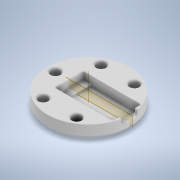
# Autodesk Inventor part: hmmb
Saved by Autodesk Inventor 2021 (Build 250183000, 183)
## iProperties
Created: 2020-07-09
Part Number: hmmb
Material: Generic
Document SubType Name: Modeling
Designer: andre
Density: 1 g/cm^3
Appearance: Default
Author: andre
## iProperties of the stored document _3DPrint.ipt
Created: 2020-07-09
Part Number: _3DPrint
Material: Generic
Document SubType Name: Modeling
Designer: andre
Density: 1 g/cm^3
Appearance: Default
Author: andre
Autodesk Inventor part; units mm, degrees
ref_plane "YZ Plane" through (0, 0, 0) normal (1, 0, 0) x (0, 1, 0)
ref_plane "XZ Plane" through (0, 0, 0) normal (0, 1, 0) x (-1, 0, 0)
ref_plane "XY Plane" through (0, 0, 0) normal (0, 0, 1) x (1, 0, 0)
sketch "Sketch1" plane through (0, 0, 0) normal (0, 1, 0) x (-1, 0, 0)
  circle A0 centre (0, 0) radius 26
  dimension "d0" = 52
  constraints: 1 centre point
  measures "d0" diameter of A0
extrude "Extrusion1" add sketch "Sketch1" along normal blind 8
chamfer "Chamfer2" distance 1.6 angle 45 1 edges at (26, 0, 0)
sketch "Sketch2" plane through (0, 8, 0) normal (0, 1, 0) x (1, 0, 0)
  line L0 (-12.4, -8.99) -> (23.96, -8.99)
  line L1 (23.96, -8.99) -> (23.96, 8.99)
  line L2 (23.96, 8.99) -> (-12.4, 8.99)
  line L3 (-12.4, 8.99) -> (-12.4, -8.99)
  point P0 (0, 0)
  dimension "d5" = 36.36
  dimension "d6" = 17.98
  dimension "d7" = 8.99
  dimension "d8" = 12.4
  constraints: 8 end point, 2 parallel, 1 horizontal, 1 perpendicular
  measures "d5" distance of L2.end L1.end
  measures "d6" distance of L1.end L0.end
  measures "d7" distance from line of point (0, 0) L2
  measures "d8" distance from line of point (0, 0) L3
extrude "Extrusion2" cut sketch "Sketch2" against normal blind 4.8
sketch "Sketch3" plane through (23.96, 8, -8.99) normal (-1, 0, 0) x (0, 0, 1)
  line L0 (4, 0) -> (13.98, 0)
  line L1 (13.98, 0) -> (13.98, -3.8)
  line L2 (13.98, -3.8) -> (4, -3.8)
  line L3 (4, -3.8) -> (4, 0)
  line L4 (0, 0) -> (17.98, 0) projected
  line L5 (0, -4.8) -> (17.98, -4.8) projected
  line L6 (0, 0) -> (0, -4.8) projected
  line L7 (17.98, 0) -> (17.98, -4.8) projected
  point P0 (8.99, -8)
  dimension "d11" = 0
  dimension "d14" = 4
  dimension "d44" = 4
  dimension "d47" = 1
  constraints: 8 end point, 2 parallel, 1 horizontal, 1 perpendicular
  measures "d11" distance between parallel lines of L4 L0
  measures "d14" distance between parallel lines of L7 L1
  measures "d44" distance between parallel lines of L6 L3
  measures "d47" distance between parallel lines of L5 L2
extrude "Extrusion3" cut sketch "Sketch3" against normal through all contours L0 L1 L2 L3
ref_plane "Work Plane1" through (-12.4, 8, 0) normal (0, 0, 1) x (1, 0, 0)
sketch "Sketch7" plane through (0, 3.2, 0) normal (0, 1, 0) x (1, 0, 0)
  line L0 (-7.4, 8.99) -> (21.36, 8.99)
  line L1 (21.36, 8.99) -> (21.36, -8.99)
  line L2 (21.36, -8.99) -> (-7.4, -8.99)
  line L3 (-7.4, -8.99) -> (-7.4, 8.99)
  line L4 (36.4, 0) -> (-36.4, 0) projected
  line L5 (-12.4, -8.99) -> (-12.4, 8.99) projected
  line L6 (23.96, -8.99) -> (-12.4, -8.99) projected
  line L7 (23.96, -4.99) -> (23.96, -8.99) projected
  line L8 (-12.4, 8.99) -> (23.96, 8.99) projected
  point P0 (0, 0)
  dimension "d31" = 5
  dimension "d98" = 2.6
  dimension "d99" = 0
  dimension "d100" = 0
  constraints: 8 end point, 2 parallel, 1 horizontal, 1 perpendicular
  measures "d31" distance between parallel lines of L5 L3
  measures "d98" distance between parallel lines of L7 L1
  measures "d99" distance between parallel lines of L6 L2
  measures "d100" distance between parallel lines of L8 L0
extrude "Extrusion5" cut sketch "Sketch7" against normal blind 1.6 contours L0 L1 L4 L3 | L4 L1 L2 L3
sketch "Sketch4" plane through (0, 8, 0) normal (0, 1, 0) x (1, 0, 0)
  circle A0 centre (-21, 0) radius 2.8
  arc A1 (25.5167, 4.99) -> (25.5167, -4.99) centre (0, 0) ccw projected
  point P0 (24.6995, 8.12)
  point P1 (24.6995, -8.12)
  dimension "d17" = 5.6
  dimension "d23" = 21
  constraints: 1 centre point
  measures "d17" diameter of A0
  measures "d23" distance of A0.centre A1.centre
extrude "Extrusion4" cut sketch "Sketch4" against normal blind 5.2
fillet "Fillet4" radius 1 1 edges at (-23.8, 8, 0)
pattern_circular "Circular Pattern2" count 5 over 240 about axis through (0, 8, 0) along (0, 1, 0) of "Extrusion4", "Fillet4" both ways yes
fillet "Fillet7" radius 0.8 4 edges at (23.96, 5.6, -8.99) (23.96, 5.6, 8.99) (-12.4, 5.6, 8.99) (-12.4, 5.6, -8.99) curvature continuous yes
sketch "Sketch12" plane through (0, 0, 0) normal (0, -1, 0) x (1, 0, 0)
  line L0 (12.3547, 15) -> (12.3547, -15) construction
  line L1 (12.3547, -15) -> (-12.3547, -15) construction
  line L2 (-12.3547, -15) -> (-12.3547, 15) construction
  line L3 (-12.3547, 15) -> (12.3547, 15) construction
  spline S0 degree 2 poles (-6.9887, 11.414) (-7, 11.0864) (-6.7175, 10.6231) (-6.3785, 10.3858) knots 0 0 0 1 2 2 2
  line L4 (-6.3785, 10.3858) -> (-1.8136, 7.1542)
  line L5 (-1.8136, 7.1542) -> (-1.8136, 7.0864)
  line L6 (-1.8136, 7.0864) -> (-6.3898, 3.8321)
  spline S1 degree 2 poles (-6.3898, 3.8321) (-6.7062, 3.6061) (-7, 3.109) (-6.9887, 2.77) knots 0 0 0 1 2 2 2
  spline S2 degree 2 poles (-6.9887, 2.77) (-6.9774, 2.2615) (-6.3672, 1.5948) (-5.8814, 1.5835) knots 0 0 0 1 2 2 2
  spline S3 degree 2 poles (-5.8814, 1.5835) (-5.6554, 1.5835) (-5.2373, 1.7304) (-5.0339, 1.8886) knots 0 0 0 1 2 2 2
  line L7 (-5.0339, 1.8886) -> (-0.0395, 5.527)
  line L8 (-0.0395, 5.527) -> (0.0282, 5.527)
  line L9 (0.0282, 5.527) -> (5.113, 1.7756)
  spline S4 degree 2 poles (5.113, 1.7756) (5.3277, 1.6174) (5.7345, 1.4705) (5.9492, 1.4818) knots 0 0 0 1 2 2 2
  spline S5 degree 2 poles (5.9492, 1.4818) (6.4011, 1.4931) (6.9887, 2.1598) (6.9887, 2.657) knots 0 0 0 1 2 2 2
  spline S6 degree 2 poles (6.9887, 2.657) (7, 2.996) (6.7062, 3.4479) (6.3898, 3.6626) knots 0 0 0 1 2 2 2
  line L10 (6.3898, 3.6626) -> (1.7006, 6.9169)
  line L11 (1.7006, 6.9169) -> (1.7006, 6.9847)
  line L12 (1.7006, 6.9847) -> (6.3107, 10.1485)
  spline S7 degree 2 poles (6.3107, 10.1485) (6.6723, 10.3971) (7, 10.9056) (6.9887, 11.2446) knots 0 0 0 1 2 2 2
  spline S8 degree 2 poles (6.9887, 11.2446) (6.9887, 11.7982) (6.3559, 12.4762) (5.8588, 12.4875) knots 0 0 0 1 2 2 2
  spline S9 degree 2 poles (5.8588, 12.4875) (5.6328, 12.4875) (5.2034, 12.3519) (4.9548, 12.1598) knots 0 0 0 1 2 2 2
  line L13 (4.9548, 12.1598) -> (0.0847, 8.6231)
  line L14 (0.0847, 8.6231) -> (0.0169, 8.6231)
  line L15 (0.0169, 8.6231) -> (-5.0791, 12.2728)
  spline S10 degree 2 poles (-5.0791, 12.2728) (-5.3051, 12.431) (-5.7232, 12.5892) (-5.9266, 12.5892) knots 0 0 0 1 2 2 2
  spline S11 degree 2 poles (-5.9266, 12.5892) (-6.3898, 12.5779) (-6.9774, 11.9225) (-6.9887, 11.414) knots 0 0 0 1 2 2 2
  spline S12 degree 2 poles (-6.9887, -2.6344) (-7, -2.9621) (-6.7175, -3.4253) (-6.3785, -3.6626) knots 0 0 0 1 2 2 2
  line L16 (-6.3785, -3.6626) -> (-1.8136, -6.8943)
  line L17 (-1.8136, -6.8943) -> (-1.8136, -6.9621)
  line L18 (-1.8136, -6.9621) -> (-6.3898, -10.2163)
  spline S13 degree 2 poles (-6.3898, -10.2163) (-6.7062, -10.4423) (-7, -10.9395) (-6.9887, -11.2785) knots 0 0 0 1 2 2 2
  spline S14 degree 2 poles (-6.9887, -11.2785) (-6.9774, -11.7869) (-6.3672, -12.4536) (-5.8814, -12.4649) knots 0 0 0 1 2 2 2
  spline S15 degree 2 poles (-5.8814, -12.4649) (-5.6554, -12.4649) (-5.2373, -12.318) (-5.0339, -12.1598) knots 0 0 0 1 2 2 2
  line L19 (-5.0339, -12.1598) -> (-0.0395, -8.5214)
  line L20 (-0.0395, -8.5214) -> (0.0282, -8.5214)
  line L21 (0.0282, -8.5214) -> (5.113, -12.2728)
  spline S16 degree 2 poles (5.113, -12.2728) (5.3277, -12.431) (5.7345, -12.5779) (5.9492, -12.5666) knots 0 0 0 1 2 2 2
  spline S17 degree 2 poles (5.9492, -12.5666) (6.4011, -12.5553) (6.9887, -11.8886) (6.9887, -11.3914) knots 0 0 0 1 2 2 2
  spline S18 degree 2 poles (6.9887, -11.3914) (7, -11.0525) (6.7062, -10.6005) (6.3898, -10.3858) knots 0 0 0 1 2 2 2
  line L22 (6.3898, -10.3858) -> (1.7006, -7.1316)
  line L23 (1.7006, -7.1316) -> (1.7006, -7.0638)
  line L24 (1.7006, -7.0638) -> (6.3107, -3.8999)
  spline S19 degree 2 poles (6.3107, -3.8999) (6.6723, -3.6513) (7, -3.1429) (6.9887, -2.8039) knots 0 0 0 1 2 2 2
  spline S20 degree 2 poles (6.9887, -2.8039) (6.9887, -2.2502) (6.3559, -1.5722) (5.8588, -1.5609) knots 0 0 0 1 2 2 2
  spline S21 degree 2 poles (5.8588, -1.5609) (5.6328, -1.5609) (5.2034, -1.6965) (4.9548, -1.8886) knots 0 0 0 1 2 2 2
  line L25 (4.9548, -1.8886) -> (0.0847, -5.4253)
  line L26 (0.0847, -5.4253) -> (0.0169, -5.4253)
  line L27 (0.0169, -5.4253) -> (-5.0791, -1.7756)
  spline S22 degree 2 poles (-5.0791, -1.7756) (-5.3051, -1.6174) (-5.7232, -1.4592) (-5.9266, -1.4592) knots 0 0 0 1 2 2 2
  spline S23 degree 2 poles (-5.9266, -1.4592) (-6.3898, -1.4705) (-6.9774, -2.1259) (-6.9887, -2.6344) knots 0 0 0 1 2 2 2
  point P0 (0, 0)
  dimension "d80" = 30
  dimension "d81" = 15
  dimension "d82" = 24.7094
  dimension "d83" = 12.3547
  constraints: 2 other
  measures "d80" distance between parallel lines of L1 L3
  measures "d81" distance from line of point (0, 0) L1
  measures "d82" distance between parallel lines of L2 L0
  measures "d83" distance from line of point (0, 0) L2
extrude "Extrusion9" cut sketch "Sketch12" against normal blind 1
sketch "Sketch13" plane through (0, 0, 0) normal (0, -1, 0) x (1, 0, 0)
  line L0 (-14.251, 6.9467) -> (-14.251, -6.9467) construction
  line L1 (-14.251, -6.9467) -> (-20.3478, -6.9467) construction
  line L2 (-20.3478, -6.9467) -> (-20.3478, 6.9467) construction
  line L3 (-20.3478, 6.9467) -> (-14.251, 6.9467) construction
  line L4 (-36.4, 0) -> (36.4, 0) projected
  spline S0 degree 2 poles (-19.7994, 4.3225) (-19.7994, 4.1816) (-19.6867, 3.9883) (-19.5498, 3.8957) knots 0 0 0 1 2 2 2
  line L5 (-19.5498, 3.8957) -> (-18.0321, 2.8249)
  line L6 (-18.0321, 2.8249) -> (-18.0321, 2.8007)
  line L7 (-18.0321, 2.8007) -> (-19.5458, 1.7138)
  spline S1 degree 2 poles (-19.5458, 1.7138) (-19.6786, 1.6171) (-19.7994, 1.4078) (-19.7994, 1.2709) knots 0 0 0 1 2 2 2
  spline S2 degree 2 poles (-19.7994, 1.2709) (-19.7954, 1.0535) (-19.5458, 0.7878) (-19.3405, 0.7838) knots 0 0 0 1 2 2 2
  spline S3 degree 2 poles (-19.3405, 0.7838) (-19.2398, 0.7798) (-19.0587, 0.8482) (-18.9701, 0.9167) knots 0 0 0 1 2 2 2
  line L8 (-18.9701, 0.9167) -> (-17.3115, 2.1445)
  line L9 (-17.3115, 2.1445) -> (-17.2873, 2.1445)
  line L10 (-17.2873, 2.1445) -> (-15.6005, 0.8804)
  spline S4 degree 2 poles (-15.6005, 0.8804) (-15.5079, 0.808) (-15.3308, 0.7436) (-15.2342, 0.7436) knots 0 0 0 1 2 2 2
  spline S5 degree 2 poles (-15.2342, 0.7436) (-15.049, 0.7516) (-14.8034, 1.0334) (-14.7994, 1.2387) knots 0 0 0 1 2 2 2
  spline S6 degree 2 poles (-14.7994, 1.2387) (-14.7994, 1.3837) (-14.9202, 1.5688) (-15.049, 1.6574) knots 0 0 0 1 2 2 2
  line L11 (-15.049, 1.6574) -> (-16.6231, 2.7323)
  line L12 (-16.6231, 2.7323) -> (-16.6231, 2.7605)
  line L13 (-16.6231, 2.7605) -> (-15.0812, 3.7991)
  spline S7 degree 2 poles (-15.0812, 3.7991) (-14.9363, 3.8998) (-14.7994, 4.1171) (-14.7994, 4.2581) knots 0 0 0 1 2 2 2
  spline S8 degree 2 poles (-14.7994, 4.2581) (-14.8034, 4.4875) (-15.0691, 4.7733) (-15.2785, 4.7774) knots 0 0 0 1 2 2 2
  spline S9 degree 2 poles (-15.2785, 4.7774) (-15.3751, 4.7774) (-15.5603, 4.7089) (-15.669, 4.6284) knots 0 0 0 1 2 2 2
  line L14 (-15.669, 4.6284) -> (-17.2672, 3.4529)
  line L15 (-17.2672, 3.4529) -> (-17.2954, 3.4529)
  line L16 (-17.2954, 3.4529) -> (-18.9902, 4.6687)
  spline S10 degree 2 poles (-18.9902, 4.6687) (-19.0909, 4.7411) (-19.264, 4.8056) (-19.3566, 4.8056) knots 0 0 0 1 2 2 2
  spline S11 degree 2 poles (-19.3566, 4.8056) (-19.5458, 4.8015) (-19.7954, 4.5318) (-19.7994, 4.3225) knots 0 0 0 1 2 2 2
  spline S12 degree 2 poles (-19.7994, -1.2307) (-19.7994, -1.3716) (-19.6867, -1.5648) (-19.5498, -1.6574) knots 0 0 0 1 2 2 2
  line L17 (-19.5498, -1.6574) -> (-18.0321, -2.7283)
  line L18 (-18.0321, -2.7283) -> (-18.0321, -2.7524)
  line L19 (-18.0321, -2.7524) -> (-19.5458, -3.8394)
  spline S13 degree 2 poles (-19.5458, -3.8394) (-19.6786, -3.936) (-19.7994, -4.1453) (-19.7994, -4.2822) knots 0 0 0 1 2 2 2
  spline S14 degree 2 poles (-19.7994, -4.2822) (-19.7954, -4.4996) (-19.5458, -4.7653) (-19.3405, -4.7693) knots 0 0 0 1 2 2 2
  spline S15 degree 2 poles (-19.3405, -4.7693) (-19.2398, -4.7733) (-19.0587, -4.7049) (-18.9701, -4.6365) knots 0 0 0 1 2 2 2
  line L20 (-18.9701, -4.6365) -> (-17.3115, -3.4086)
  line L21 (-17.3115, -3.4086) -> (-17.2873, -3.4086)
  line L22 (-17.2873, -3.4086) -> (-15.6005, -4.6727)
  spline S16 degree 2 poles (-15.6005, -4.6727) (-15.5079, -4.7452) (-15.3308, -4.8096) (-15.2342, -4.8096) knots 0 0 0 1 2 2 2
  spline S17 degree 2 poles (-15.2342, -4.8096) (-15.049, -4.8015) (-14.8034, -4.5197) (-14.7994, -4.3144) knots 0 0 0 1 2 2 2
  spline S18 degree 2 poles (-14.7994, -4.3144) (-14.7994, -4.1695) (-14.9202, -3.9843) (-15.049, -3.8957) knots 0 0 0 1 2 2 2
  line L23 (-15.049, -3.8957) -> (-16.6231, -2.8209)
  line L24 (-16.6231, -2.8209) -> (-16.6231, -2.7927)
  line L25 (-16.6231, -2.7927) -> (-15.0812, -1.754)
  spline S19 degree 2 poles (-15.0812, -1.754) (-14.9363, -1.6534) (-14.7994, -1.436) (-14.7994, -1.2951) knots 0 0 0 1 2 2 2
  spline S20 degree 2 poles (-14.7994, -1.2951) (-14.8034, -1.0656) (-15.0691, -0.7798) (-15.2785, -0.7758) knots 0 0 0 1 2 2 2
  spline S21 degree 2 poles (-15.2785, -0.7758) (-15.3751, -0.7758) (-15.5603, -0.8442) (-15.669, -0.9247) knots 0 0 0 1 2 2 2
  line L26 (-15.669, -0.9247) -> (-17.2672, -2.1002)
  line L27 (-17.2672, -2.1002) -> (-17.2954, -2.1002)
  line L28 (-17.2954, -2.1002) -> (-18.9902, -0.8845)
  spline S22 degree 2 poles (-18.9902, -0.8845) (-19.0909, -0.812) (-19.264, -0.7476) (-19.3566, -0.7476) knots 0 0 0 1 2 2 2
  spline S23 degree 2 poles (-19.3566, -0.7476) (-19.5458, -0.7516) (-19.7954, -1.0213) (-19.7994, -1.2307) knots 0 0 0 1 2 2 2
  point P0 (0, 0)
  dimension "d86" = 13.8935
  dimension "d87" = 6.9467
  constraints: 2 other
  measures "d86" distance between parallel lines of L1 L3
  measures "d87" distance between parallel lines of L4 L1
extrude "Extrusion10" cut sketch "Sketch13" against normal blind 2
fillet "Fillet9" radius 2 2 edges at (24.7383, 4.2, -4.99) (24.7383, 4.2, 4.99) curvature continuous yes
equation "\"d7\" = 0.5 * d6"
equation "\"d44\" = d14"
equation "\"d81\" = 0.5 * d80"
equation "\"d83\" = 0.5 * d82"
equation "\"d24\" = 0.5 * d6"
body "Solid1"
